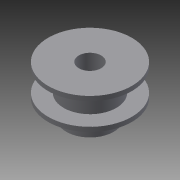
# Autodesk Inventor part: CAD:pulley_8mm
Saved by Autodesk Inventor 2015 (Build 190159000, 159)
## iProperties
Created: 2015-08-29
Material: Generic
Description: pulley 8mm
Document SubType Name: Modeling
Designer: francis
Density: 1 g/cm^3
Appearance: Default
Stock Number: RS online 778 4831
Part Category: insert part category here and press enter to fill value
Author: francis
Autodesk Inventor part; units mm, degrees
ref_plane "YZ Plane" through (0, 0, 0) normal (1, 0, 0) x (0, 1, 0)
ref_plane "XZ Plane" through (0, 0, 0) normal (0, 1, 0) x (-1, 0, 0)
ref_plane "XY Plane" through (0, 0, 0) normal (0, 0, 1) x (1, 0, 0)
sketch "Sketch1" plane through (0, 0, 0) normal (1, 0, 0) x (0, 1, 0)
  line L0 (0, 17.5) -> (11, 17.5)
  line L1 (11, 17.5) -> (11, 15.9)
  line L2 (11, 15.9) -> (5.445, 15.9)
  line L3 (5.445, 15.9) -> (5.445, 7.9)
  line L4 (5.445, 7.9) -> (11, 7.9)
  line L5 (11, 7.9) -> (11, 6.3)
  line L6 (11, 6.3) -> (4.5, 6.3)
  line L7 (4.5, 6.3) -> (4.5, 0)
  line L8 (4.5, 0) -> (0, 0)
  line L9 (0, 0) -> (0, 17.5)
  line L10 (-4, 10.0812) -> (-4, 1.7277) construction
  dimension "d0" = 30
  dimension "d1" = 17.5
  dimension "d2" = 8
  dimension "d3" = 11.2
  dimension "d4" = 8
  dimension "d5" = 17
  dimension "d6" = 18.89
  constraints: 22 end point, 8 perpendicular, 2 point on line, 1 collinear, 1 horizontal, 1 vertical
  measures "d0" diameter of L1 L10
  measures "d1" distance between parallel lines of L0 L8
  measures "d2" distance between parallel lines of L4 L2
  measures "d3" distance between parallel lines of L0 L6
  measures "d4" diameter of L9 L10
  measures "d5" diameter of L7 L10
  measures "d6" diameter of L3 L10
revolve "Revolution1" add sketch "Sketch1" angle 360 about axis through (0, -4, 10.0812) along (0, 0, -1)
sketch "Sketch2" plane through (0, 0, 0) normal (1, 0, 0) x (0, 1, 0)
  line L0 (-12.5, 6.3) -> (-12.5, 0) construction
  line L1 (4.5, 6.3) -> (4.5, 0) construction
  line L2 (-12.5, 0) -> (4.5, 0) construction
  line L3 (-11.6, 0) -> (6.6, 0) construction
  point P0 (0, 0)
  point P1 (-2.5, 3)
  point P2 (-2.5, 3)
  dimension "d8" = 3
  constraints: 1 coincident
  measures "d8" distance from line of L2 point (-2.5, 3)
hole "Hole1" at (0, -2.5, 3) direction (-1, 0, 0) diameter 2.459 end through all thread size "M3x0.5" class "6H" standard "ISO Metric profile"
body "Solid1"
